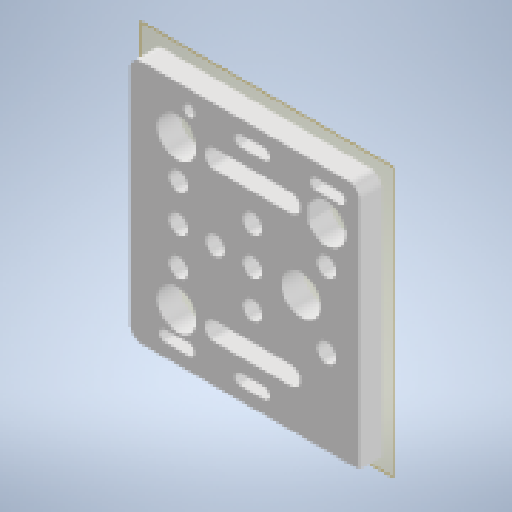
# Autodesk Inventor part: фанера жесть
Saved by Autodesk Inventor 2024.2 (Build 282272000, 272)
## iProperties
Created: 2026-02-11
Part Number: фанера жесть
Material: Типовые
Document SubType Name: Modeling
Designer: katya_notebook
Density: 1 g/cm^3
Appearance: По умолчанию
Author: katya_notebook
Autodesk Inventor part; units mm, degrees
ref_plane "YZ Plane" through (0, 0, 0) normal (1, 0, 0) x (0, 1, 0)
ref_plane "XZ Plane" through (0, 0, 0) normal (0, 1, 0) x (-1, 0, 0)
ref_plane "XY Plane" through (0, 0, 0) normal (0, 0, 1) x (1, 0, 0)
ref_plane "РабПлоскость1" through (0, 0, 0) normal (0, 0, 1) x (1, 0, 0)
sketch "Эскиз1" plane through (0, 0, 0) normal (0, 0, 1) x (1, 0, 0)
  circle A0 centre (-9.825, -4) radius 5.25 projected
  circle A1 centre (-39.775, 23.7) radius 1.5 projected
  circle A2 centre (-43.025, 16) radius 5.25 projected
  circle A3 centre (-43.025, -24) radius 5.25 projected
  arc A4 (-37.417, -36.75) -> (-33.544, -33.75) centre (-37.417, -32.75) ccw projected
  line L0 (-33.544, -33.75) -> (-9.875, -33.75) projected
  arc A5 (-9.875, -33.75) -> (-7.875, -31.75) centre (-9.875, -31.75) ccw projected
  line L1 (-7.875, -31.75) -> (-7.875, -21.99) projected
  arc A6 (0.7295, -20.3304) -> (-7.875, -21.99) centre (-3.025, -24) ccw projected
  arc A7 (0.7295, -20.3304) -> (5.875, -18.2335) centre (2.875, -18.2335) ccw projected
  line L2 (5.875, -18.2335) -> (5.875, 25.75) projected
  arc A8 (5.875, 25.75) -> (2.875, 28.75) centre (2.875, 25.75) ccw projected
  line L3 (2.875, 28.75) -> (-52.625, 28.75) projected
  arc A9 (-52.625, 28.75) -> (-55.625, 25.75) centre (-52.625, 25.75) ccw projected
  line L4 (-55.625, 25.75) -> (-55.625, -33.75) projected
  arc A10 (-55.625, -33.75) -> (-52.625, -36.75) centre (-52.625, -33.75) ccw projected
  line L5 (-52.625, -36.75) -> (-37.417, -36.75) projected
  arc A11 (-39.775, -33.2) -> (-39.775, -30.2) centre (-39.775, -31.7) ccw projected
  line L6 (-39.775, -33.2) -> (-46.275, -33.2) projected
  arc A12 (-46.275, -30.2) -> (-46.275, -33.2) centre (-46.275, -31.7) ccw projected
  line L7 (-46.275, -30.2) -> (-39.775, -30.2) projected
  line L8 (-7.875, 13.99) -> (-7.875, 18.01) projected
  arc A13 (-7.875, 13.99) -> (-7.875, 18.01) centre (-3.025, 16) ccw projected
  arc A14 (-33.195, 18.5) -> (-33.195, 13.5) centre (-33.195, 16) ccw projected
  line L9 (-33.195, 18.5) -> (-12.555, 18.5) projected
  arc A15 (-12.555, 13.5) -> (-12.555, 18.5) centre (-12.555, 16) ccw projected
  line L10 (-12.555, 13.5) -> (-33.195, 13.5) projected
  line L11 (-26.125, -30.2) -> (-19.625, -30.2) projected
  arc A16 (-19.625, -33.2) -> (-19.625, -30.2) centre (-19.625, -31.7) ccw projected
  line L12 (-19.625, -33.2) -> (-26.125, -33.2) projected
  arc A17 (-26.125, -30.2) -> (-26.125, -33.2) centre (-26.125, -31.7) ccw projected
  circle A18 centre (-22.875, 6) radius 2.55 projected
  circle A19 centre (-22.875, -4) radius 2.55 projected
  circle A20 centre (-22.875, -14) radius 2.55 projected
  circle A21 centre (-32.875, -4) radius 2.55 projected
  arc A22 (-12.555, -26.5) -> (-12.555, -21.5) centre (-12.555, -24) ccw projected
  line L13 (-12.555, -26.5) -> (-33.195, -26.5) projected
  arc A23 (-33.195, -21.5) -> (-33.195, -26.5) centre (-33.195, -24) ccw projected
  line L14 (-33.195, -21.5) -> (-12.555, -21.5) projected
  line L15 (-26.125, 25.2) -> (-19.625, 25.2) projected
  arc A24 (-19.625, 22.2) -> (-19.625, 25.2) centre (-19.625, 23.7) ccw projected
  line L16 (-19.625, 22.2) -> (-26.125, 22.2) projected
  arc A25 (-26.125, 25.2) -> (-26.125, 22.2) centre (-26.125, 23.7) ccw projected
  circle A26 centre (-42.725, -4) radius 2.55 projected
  circle A27 centre (-42.725, 6) radius 2.55 projected
  circle A28 centre (-42.725, -14) radius 2.55 projected
  arc A29 (-5.875, 25.2) -> (-5.875, 22.2) centre (-5.875, 23.7) ccw projected
  line L17 (-5.875, 25.2) -> (0.525, 25.2) projected
  arc A30 (0.525, 22.2) -> (0.525, 25.2) centre (0.525, 23.7) ccw projected
  line L18 (0.525, 22.2) -> (-5.875, 22.2) projected
  circle A31 centre (-3.025, 6) radius 2.55 projected
  circle A32 centre (-3.025, -14) radius 2.55 projected
  line L19 (-37.417, -36.75) -> (-9.875, -36.75)
  line L20 (-9.875, -36.75) -> (-9.875, -31.75)
  line L21 (-9.875, -33.75) -> (-7.875, -33.75)
  line L22 (-7.875, -33.75) -> (-7.875, -31.75)
  line L23 (-9.875, -36.75) -> (-7.875, -36.75)
  line L24 (-7.875, -36.75) -> (-7.875, -33.75)
  point P0 (0, 0)
  constraints: 12 end point, 3 horizontal, 1 collinear, 1 perpendicular, 1 point on line
extrude "Выдавливание1" add sketch "Эскиз1" along normal blind 6
fillet "Сопряжение1" radius 8 1 edges at (-7.875, -36.75, 3)
